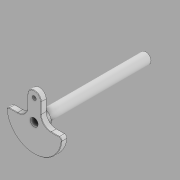
# Autodesk Inventor part: CrankShaft
Saved by Autodesk Inventor 2020 (Build 240168000, 168)
## iProperties
Created: 2019-10-15
Part Number: CrankShaft
Material: Genérico
Document SubType Name: Modeling
Designer: gerar
Density: 1 g/cm^3
Appearance: Valor por defecto
Author: Gerardo Naranjo
Title: CrankShaft
Autodesk Inventor part; units mm, degrees
ref_plane "YZ Plane" through (0, 0, 0) normal (1, 0, 0) x (0, 1, 0)
ref_plane "XZ Plane" through (0, 0, 0) normal (0, 1, 0) x (-1, 0, 0)
ref_plane "XY Plane" through (0, 0, 0) normal (0, 0, 1) x (1, 0, 0)
sketch "Boceto1" plane through (0, 0, 0) normal (0, 0, 1) x (1, 0, 0)
  circle A0 centre (0, 0) radius 2.3813
  arc A1 (4.0409, 12.7) -> (-4.0409, 12.7) centre (0, 12.7) ccw
  arc A2 (-10.1023, 0) -> (-4.0409, 6.0614) centre (-10.1023, 6.0614) ccw
  line L0 (-4.0409, 12.7) -> (-4.0409, 6.0614)
  line L1 (4.0409, 12.7) -> (4.0409, 6.0614)
  arc A3 (4.0409, 6.0614) -> (10.1023, 0) centre (10.1023, 6.0614) ccw
  arc A4 (-15.0775, 0) -> (-16.5852, -1.6669) centre (-15.0775, -1.5153) ccw
  line L2 (-23.7372, 0) -> (23.7372, 0) construction
  arc A5 (16.5852, -1.6669) -> (15.0775, 0) centre (15.0775, -1.5153) ccw
  arc A6 (-16.5852, -1.6669) -> (16.5852, -1.6669) centre (0, 0) ccw
  line L3 (10.1023, 0) -> (15.0775, 0)
  line L4 (-15.0775, 0) -> (-10.1023, 0)
  dimension "d1" = 4.7625
  dimension "d2" = 8.0818
  dimension "d3" = 12.1227
  dimension "d5" = 12.7
  dimension "d6" = 3.0307
  constraints: 12 point on circle, 10 tangent, 8 end point, 7 centre point, 4 point on line, 2 coincident, 2 equal radius, 2 horizontal, 2 vertical
  measures "d1" diameter of A0
  measures "d2" diameter of A1
  measures "d3" diameter of A2
  measures "d5" distance of point (0, 0) A1.centre
  measures "d6" diameter of A4
extrude "Extrusión1" add sketch "Boceto1" against normal blind 3.175
sketch "Boceto2" plane through (0, 0, 0) normal (0, 0, 1) x (1, 0, 0)
  line L0 (0, 0) -> (0, 12.7) construction
  line L1 (0, 0) -> (12.7, 0) construction
  dimension "d9" = 12.7
  dimension "d10" = 90
  constraints: 4 end point, 1 coincident, 1 horizontal, 1 perpendicular, 1 vertical
  measures "d9" distance of L0.start L0.end
  measures "d10" angle of L1 L0
hole "Agujero1" at (0, 12.7, 0) direction (0, 0, -1) diameter 2.4867 end through all thread size "5-40 UNC" class "2B" standard "ANSI Unified Screw Threads"
sketch "Boceto3" plane through (0, 0, -3.175) normal (0, 0, -1) x (-1, 0, 0)
  circle A0 centre (0, 0) radius 4.7625
  circle A1 centre (0, 0) radius 2.3813
  dimension "d18" = 9.525
  dimension "d19" = 4.7625
  constraints: 2 centre point, 2 coincident
  measures "d18" diameter of A0
  measures "d19" diameter of A1
extrude "Extrusión2" add sketch "Boceto3" along normal blind 2.3813
sketch "Boceto4" plane through (0, 0, -5.5563) normal (0, 0, -1) x (-1, 0, 0)
  circle A0 centre (0, 0) radius 3.175
  dimension "d22" = 6.35
  constraints: 1 centre point, 1 coincident
  measures "d22" diameter of A0
extrude "Extrusión3" add sketch "Boceto4" along normal blind 61.9125
fillet "Empalme1" radius 0.254 10 edges at (-4.0409, 9.3807, 0) (-5.8162, 1.7753, 0) (-12.5899, 0, 0) (-16.2013, -0.4988, 0) (0, -16.6688, 0) (16.2013, -0.4988, 0) (12.5899, 0, 0) (5.8162, 1.7753, 0) (4.0409, 9.3807, 0) (0, 16.7409, 0)
